Autodesk Fusion 360 part; units mm, degrees
(part 4 of 4)
sketch "Sketch1 (5)" plane through (0, -0.5, 0) normal (0, -1, 0) x (1, 0, 0) in component "Standoff"
  line L0 (9, -29.5) -> (9, -33.5)
  line L1 (9, -33.5) -> (5, -33.5)
  line L2 (5, -33.5) -> (5, -29.5)
  line L3 (5, -29.5) -> (9, -29.5)
  line L4 (53, -29.5) -> (53, -33.5)
  line L5 (53, -33.5) -> (45, -33.5)
  line L6 (45, -33.5) -> (45, -29.5)
  line L7 (45, -29.5) -> (53, -29.5)
  line L8 (84.5, 47) -> (84.5, 43.5)
  line L9 (84.5, 43.5) -> (80, 43.5)
  line L10 (80, 43.5) -> (80, 47)
  line L11 (80, 47) -> (84.5, 47)
  line L12 (53, 47) -> (53, 43.5)
  line L13 (53, 43.5) -> (45, 43.5)
  line L14 (45, 43.5) -> (45, 47)
  line L15 (45, 47) -> (53, 47)
  line L16 (84.5, -43.5) -> (84.5, -47)
  line L17 (84.5, -47) -> (80, -47)
  line L18 (80, -47) -> (80, -43.5)
  line L19 (80, -43.5) -> (84.5, -43.5)
  line L20 (12, -35.5) -> (12, -45)
  line L21 (12, -45) -> (9, -45)
  line L22 (9, -45) -> (9, -35.5)
  line L23 (9, -35.5) -> (12, -35.5)
  line L24 (26.5, 33.5) -> (26.5, 29.5)
  line L25 (26.5, 29.5) -> (20.5, 29.5)
  line L26 (20.5, 29.5) -> (20.5, 33.5)
  line L27 (20.5, 33.5) -> (26.5, 33.5)
  line L28 (53, -43.5) -> (53, -47)
  line L29 (53, -47) -> (45, -47)
  line L30 (45, -47) -> (45, -43.5)
  line L31 (45, -43.5) -> (53, -43.5)
  line L32 (84.5, 33.5) -> (84.5, 29.5)
  line L33 (84.5, 29.5) -> (78.5, 29.5)
  line L34 (78.5, 29.5) -> (78.5, 33.5)
  line L35 (78.5, 33.5) -> (84.5, 33.5)
  line L36 (53, 33.5) -> (53, 22.5)
  line L37 (53, 22.5) -> (45, 22.5)
  line L38 (45, 22.5) -> (45, 33.5)
  line L39 (45, 33.5) -> (53, 33.5)
  line L40 (84.5, -29.5) -> (84.5, -33.5)
  line L41 (84.5, -33.5) -> (78.5, -33.5)
  line L42 (78.5, -33.5) -> (78.5, -29.5)
  line L43 (78.5, -29.5) -> (84.5, -29.5)
  line L44 (23.5, -29.5) -> (26.5, -29.5)
  line L45 (26.5, -29.5) -> (26.5, -47)
  line L46 (26.5, -47) -> (23.5, -47)
  line L47 (23.5, -47) -> (23.5, -29.5)
  line L48 (9, 33.5) -> (9, 22.5)
  line L49 (9, 22.5) -> (5, 22.5)
  line L50 (5, 22.5) -> (5, 33.5)
  line L51 (5, 33.5) -> (9, 33.5)
  line L52 (76.5, -20.1237) -> (76.5, -30.9468)
  line L53 (76.5, -30.9468) -> (63.73, -44.9205)
  line L54 (63.73, -44.9205) -> (63.73, -47)
  line L55 (63.73, -47) -> (55, -47)
  line L56 (55, -47) -> (55, -21.5041)
  line L57 (55, -21.5041) -> (76.5, -20.1237)
  line L58 (76.5, -18.1196) -> (55, -19.5)
  line L59 (55, -19.5) -> (55, -1)
  line L60 (55, -1) -> (76.5, -1)
  line L61 (76.5, -1) -> (76.5, -18.1196)
  line L62 (18.5, -21.5) -> (18.5, -33.5)
  line L63 (18.5, -33.5) -> (11, -33.5)
  line L64 (11, -33.5) -> (11, -21.5)
  line L65 (11, -21.5) -> (18.5, -21.5)
  line L66 (18.5, -19.5) -> (11, -19.5)
  line L67 (11, -19.5) -> (11, -1)
  line L68 (11, -1) -> (18.5, -1)
  line L69 (18.5, -1) -> (18.5, -19.5)
  line L70 (11, 21.5) -> (11, 33.5)
  line L71 (11, 33.5) -> (18.5, 33.5)
  line L72 (18.5, 33.5) -> (18.5, 21.5)
  line L73 (18.5, 21.5) -> (11, 21.5)
  line L74 (55, 14.6033) -> (55, 47)
  line L75 (55, 47) -> (59.7352, 47)
  line L76 (59.7352, 47) -> (76.5, 39.9438)
  line L77 (76.5, 39.9438) -> (76.5, 21.6033)
  line L78 (76.5, 21.6033) -> (55, 14.6033)
  line L79 (55, 12.5) -> (76.5, 19.5)
  line L80 (76.5, 19.5) -> (76.5, 1)
  line L81 (76.5, 1) -> (55, 1)
  line L82 (55, 1) -> (55, 12.5)
  line L83 (43, -21.5) -> (43, -47)
  line L84 (43, -47) -> (28.5, -47)
  line L85 (28.5, -47) -> (28.5, -21.5)
  line L86 (28.5, -21.5) -> (43, -21.5)
  line L87 (43, -19.5) -> (28.5, -19.5)
  line L88 (28.5, -19.5) -> (28.5, -1)
  line L89 (28.5, -1) -> (43, -1)
  line L90 (43, -1) -> (43, -19.5)
  line L91 (95, -20.1196) -> (95, -47)
  line L92 (95, -47) -> (86.5, -47)
  line L93 (86.5, -47) -> (86.5, -20.1196)
  line L94 (86.5, -20.1196) -> (95, -20.1196)
  line L95 (28.5, 21.7209) -> (28.5, 47)
  line L96 (28.5, 47) -> (43, 47)
  line L97 (43, 47) -> (43, 14.7209)
  line L98 (43, 14.7209) -> (28.5, 21.7209)
  line L99 (28.5, 19.5) -> (43, 12.5)
  line L100 (43, 12.5) -> (43, 1)
  line L101 (43, 1) -> (28.5, 1)
  line L102 (28.5, 1) -> (28.5, 19.5)
  line L103 (26.5, 19.5) -> (26.5, 1)
  line L104 (26.5, 1) -> (20.5, 1)
  line L105 (20.5, 1) -> (20.5, 19.5)
  line L106 (20.5, 19.5) -> (26.5, 19.5)
  line L107 (11, 19.5) -> (18.5, 19.5)
  line L108 (18.5, 19.5) -> (18.5, 1)
  line L109 (18.5, 1) -> (11, 1)
  line L110 (11, 1) -> (11, 19.5)
  line L111 (9, 12.5) -> (9, 1)
  line L112 (9, 1) -> (5, 1)
  line L113 (5, 1) -> (5, 12.5)
  line L114 (5, 12.5) -> (9, 12.5)
  line L115 (5, -1) -> (9, -1)
  line L116 (9, -1) -> (9, -19.5)
  line L117 (9, -19.5) -> (5, -19.5)
  line L118 (5, -19.5) -> (5, -1)
  line L119 (20.5, -19.5) -> (20.5, -1)
  line L120 (20.5, -1) -> (26.5, -1)
  line L121 (26.5, -1) -> (26.5, -19.5)
  line L122 (26.5, -19.5) -> (20.5, -19.5)
  line L123 (45, -19.5) -> (45, -1)
  line L124 (45, -1) -> (53, -1)
  line L125 (53, -1) -> (53, -19.5)
  line L126 (53, -19.5) -> (45, -19.5)
  line L127 (78.5, -18.1196) -> (78.5, -1)
  line L128 (78.5, -1) -> (84.5, -1)
  line L129 (84.5, -1) -> (84.5, -18.1196)
  line L130 (84.5, -18.1196) -> (78.5, -18.1196)
  line L131 (95, -18.1196) -> (86.5, -18.1196)
  line L132 (86.5, -18.1196) -> (86.5, -1)
  line L133 (86.5, -1) -> (95, -1)
  line L134 (95, -1) -> (95, -18.1196)
  line L135 (78.5, 19.5) -> (84.5, 19.5)
  line L136 (84.5, 19.5) -> (84.5, 1)
  line L137 (84.5, 1) -> (78.5, 1)
  line L138 (78.5, 1) -> (78.5, 19.5)
  line L139 (53, 12.5) -> (53, 1)
  line L140 (53, 1) -> (45, 1)
  line L141 (45, 1) -> (45, 12.5)
  line L142 (45, 12.5) -> (53, 12.5)
  line L143 (95, 1) -> (86.5, 1)
  line L144 (86.5, 1) -> (86.5, 19.5)
  line L145 (86.5, 19.5) -> (95, 19.5)
  line L146 (95, 19.5) -> (95, 1)
  line L147 (95, 21.5) -> (86.5, 21.5)
  line L148 (86.5, 21.5) -> (86.5, 47)
  line L149 (86.5, 47) -> (95, 47)
  line L150 (95, 47) -> (95, 21.5)
  circle A0 centre (68.73, 48.639) radius 1.35
  circle A1 centre (4.33, -46.861) radius 1.35
  circle A2 centre (2.838, 46.861) radius 1.35
  circle A3 centre (68.73, -46.861) radius 1.35
  line L151 (100, 52) -> (15, 52)
  line L152 (15, 52) -> (15, 50)
  line L153 (15, 50) -> (0, 50)
  line L154 (0, 50) -> (0, -50)
  line L155 (0, -50) -> (15, -50)
  line L156 (15, -50) -> (15, -52)
  line L157 (15, -52) -> (100, -52)
  line L158 (100, -52) -> (100, 52)
  circle A4 centre (23.5, -24.5) radius 1.35
  circle A5 centre (23.5, 24.5) radius 1.35
  circle A6 centre (81.5, -24.5) radius 1.35
  circle A7 centre (81.5, 24.5) radius 1.35
  circle A8 centre (75, -46) radius 1.35
  circle A9 centre (17, 46) radius 1.35
  circle A10 centre (17, -46) radius 1.35
  circle A11 centre (75, 46) radius 1.35
  circle A12 centre (81.5, -38.5) radius 1.35
  circle A13 centre (50, 38.5) radius 1.35
  circle A14 centre (81.5, 38.5) radius 1.35
  circle A15 centre (50, -38.5) radius 1.35
  circle A16 centre (4, 38.5) radius 1.35
  circle A17 centre (4, -38.5) radius 1.35
  arc A18 (17.1594, -38.6594) -> (18.3406, -39.8406) centre (17, -40) ccw
  arc A19 (18.3406, -39.8406) -> (17.1594, -38.6594) centre (18.5, -38.5) ccw
  circle A20 centre (18.5, 38.5) radius 1.35
  circle A21 centre (6, -24.5) radius 1.35
  circle A22 centre (6, 17.5) radius 1.35
  circle A23 centre (48, -24.5) radius 1.35
  circle A24 centre (48, 17.5) radius 1.35
  circle A25 centre (75, -40) radius 1.35
  circle A26 centre (2.838, 46.861) radius 1.3
  circle A27 centre (2.838, 46.861) radius 2.45
  dimension "d415" = 2.6
  dimension "d416" = 4.9
  constraint concentric A2 A26
  constraint concentric A2 A27
  measures "d415" diameter of A26
  measures "d416" diameter of A27
extrude "Extrude2''''" add sketch "Sketch1 (5)" along normal blind 5.5 separate body contours A2 | A27 makes body 12 in component "Standoff"
component "Card Plate" placed x (1, 0, 0) y (0, 1, 0) z (0, 0, 1) at (0, 0, 0)
component "Bay Body" placed x (1, 0, 0) y (0, 1, 0) z (0, 0, 1) at (0, 0, 0)
component "End Frame A" placed x (1, 0, 0) y (0, 1, 0) z (0, 0, 1) at (0, 0, 0)
component "Standoff for End Frame" placed x (1, 0, 0) y (0, 1, 0) z (0, 0, 1) at (0, 0, 0)
component "Bay Cover" placed x (1, 0, 0) y (0, 1, 0) z (0, 0, 1) at (0, 0, 0)
component "Spacer 40 mm" placed x (1, 0, 0) y (0, 1, 0) z (0, 0, 1) at (0, 0, 0)
component "End Frame B" placed x (1, 0, 0) y (0, 1, 0) z (0, 0, 1) at (0, 0, 0)
component "Spacer 35 mm" placed x (1, 0, 0) y (0, 1, 0) z (0, 0, 1) at (0, 0, 0)
component "Standoff" placed x (1, 0, 0) y (0, 1, 0) z (0, 0, 1) at (0, 0, 0)
equation "d30 = d29"
equation "d192 = d191"
equation "d193 = d191"
equation "d194 = d191"
equation "d204 = d203"
equation "d205 = d203"
equation "d206 = d203"
equation "d207 = d203"
equation "d208 = d203"
equation "d225 = d224"
equation "d226 = d224"
equation "d227 = d224"
equation "d250 = d249"
equation "d251 = d249"
equation "d252 = d249"
